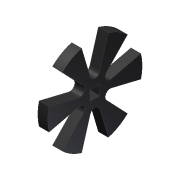
# Autodesk Inventor part: IntakeRoller
Saved by Autodesk Inventor 2012 (Build 160160000, 160)
## iProperties
Created: 2013-01-26
Part Number: IntakeRoller
Material: Silicone
Document SubType Name: Modeling
Designer: JesseK
Density: 1.25 g/cm^3
Mass: 87.6718 g
Surface Area: 210.22 cm^2
Volume: 70.1375 cm^3
Author: JesseK
Autodesk Inventor part; units mm, degrees
ref_plane "YZ Plane" through (0, 0, 0) normal (1, 0, 0) x (0, 1, 0)
ref_plane "XZ Plane" through (0, 0, 0) normal (0, 1, 0) x (-1, 0, 0)
ref_plane "XY Plane" through (0, 0, 0) normal (0, 0, 1) x (1, 0, 0)
sketch "Sketch1" plane through (0, 0, 0) normal (1, 0, 0) x (0, 1, 0)
  circle A0 centre (0, 0) radius 60.325
  line L0 (-6.35, 6.35) -> (6.35, 6.35)
  line L1 (6.35, 6.35) -> (6.35, -6.35)
  line L2 (6.35, -6.35) -> (-6.35, -6.35)
  line L3 (-6.35, -6.35) -> (-6.35, 6.35)
  line L4 (-6.35, 6.35) -> (0, 0) construction
  line L5 (0, 0) -> (6.35, 6.35) construction
  line L6 (-6.35, -6.35) -> (0, 0) construction
  line L7 (0, 0) -> (6.35, -6.35) construction
  dimension "d0" = 120.65
  dimension "d1" = 12.7
  constraints: 16 end point, 4 perpendicular, 2 parallel, 1 centre point, 1 coincident, 1 horizontal
  measures "d0" diameter of A0
  measures "d1" distance of L2.end L0.start
extrude "Extrusion1" add sketch "Sketch1" along normal blind 12.7
sketch "Sketch2" plane through (12.7, 0, 0) normal (1, 0, 0) x (0, 0, -1)
  circle A0 centre (0, 0) radius 60.325 projected
  line L0 (0, 0) -> (0, 60.325) construction
  line L1 (0, 60.325) -> (-17.056, 57.8636) construction
  line L2 (0, 60.325) -> (17.056, 57.8636) construction
  line L3 (17.056, 57.8636) -> (0, 0) construction
  line L4 (0, 0) -> (-17.056, 57.8636) construction
  arc A1 (17.056, 57.8636) -> (-17.056, 57.8636) centre (0, 0) ccw construction
  line L5 (-17.056, 57.8636) -> (-1.4908, 15.3294)
  line L6 (1.4908, 15.3294) -> (17.056, 57.8636)
  arc A2 (-1.4908, 15.3294) -> (1.4908, 15.3294) centre (0, 15.875) ccw
  dimension "d4" = 32.847
  dimension "d11" = 1.5875
  dimension "d12" = 44.45
  constraints: 14 end point, 9 point on circle, 2 centre point, 2 equal length, 2 tangent, 1 coincident, 1 point on line, 1 vertical
  measures "d4" angle of L3 L4
  measures "d11" radius of A2
  measures "d12" distance of L0.end A2.centre
extrude "Extrusion3" cut sketch "Sketch2" against normal through all contours L6 A2 L5 A0 picked at (-9.0544, 44.2998)
pattern_circular "Circular Pattern2" count 10 over 360 about axis through (0, 0, 0) along (1, 0, 0) of "Extrusion3"
body "Solid1"
